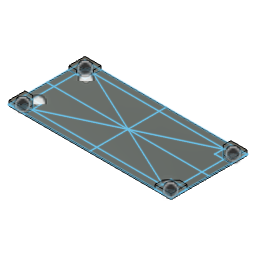
pcb_mount (Autodesk Fusion 360 design; units mm, degrees)
Autodesk Fusion 360 part; units mm, degrees
sketch "Sketch1" plane through (0, 0, 0) normal (0, 0, 1) x (1, 0, 0)
  line L0 (-1.15, -7.9615) -> (94.86, -7.9615)
  line L1 (94.86, -7.9615) -> (94.86, -52.9715)
  line L2 (94.86, -52.9715) -> (-1.15, -52.9715)
  line L3 (-1.15, -52.9715) -> (-1.15, -7.9615)
  line L4 (3, -11.9865) -> (90.71, -11.9865)
  line L5 (90.71, -11.9865) -> (90.71, -48.9465)
  line L6 (90.71, -48.9465) -> (3, -48.9465)
  line L7 (3, -48.9465) -> (3, -11.9865)
  line L8 (-1.15, -7.9615) -> (94.86, -52.9715)
  line L9 (94.86, -7.9615) -> (-1.15, -52.9715)
  line L10 (46.855, -30.4665) -> (46.855, -7.9615)
  line L11 (46.855, -30.4665) -> (46.855, -52.9715)
  line L12 (46.855, -30.4665) -> (94.86, -30.4665)
  line L13 (46.855, -30.4665) -> (-1.15, -30.4665)
  circle A0 centre (3, -11.9865) radius 1.55
  circle A1 centre (3, -48.9465) radius 1.55
  circle A2 centre (90.71, -48.9465) radius 1.55
  circle A3 centre (90.71, -11.9865) radius 1.55
  line L14 (6.2324, -12.0561) -> (4.6765, -9.2219)
  line L15 (4.6765, -9.2219) -> (1.4441, -9.1523)
  line L16 (1.4441, -9.1523) -> (-0.2324, -11.9168)
  line L17 (-0.2324, -11.9168) -> (1.3235, -14.751)
  line L18 (1.3235, -14.751) -> (4.5559, -14.8206)
  line L19 (4.5559, -14.8206) -> (6.2324, -12.0561)
  line L20 (4.6166, -51.7465) -> (6.2332, -48.9465)
  line L21 (6.2332, -48.9465) -> (4.6166, -46.1465)
  line L22 (4.6166, -46.1465) -> (1.3834, -46.1465)
  line L23 (1.3834, -46.1465) -> (-0.2332, -48.9465)
  line L24 (-0.2332, -48.9465) -> (1.3834, -51.7465)
  line L25 (1.3834, -51.7465) -> (4.6166, -51.7465)
  line L26 (92.3266, -51.7465) -> (93.9432, -48.9465)
  line L27 (93.9432, -48.9465) -> (92.3266, -46.1465)
  line L28 (92.3266, -46.1465) -> (89.0934, -46.1465)
  line L29 (89.0934, -46.1465) -> (87.4768, -48.9465)
  line L30 (87.4768, -48.9465) -> (89.0934, -51.7465)
  line L31 (89.0934, -51.7465) -> (92.3266, -51.7465)
  line L32 (92.3266, -14.7865) -> (93.9432, -11.9865)
  line L33 (93.9432, -11.9865) -> (92.3266, -9.1865)
  line L34 (92.3266, -9.1865) -> (89.0934, -9.1865)
  line L35 (89.0934, -9.1865) -> (87.4768, -11.9865)
  line L36 (87.4768, -11.9865) -> (89.0934, -14.7865)
  line L37 (89.0934, -14.7865) -> (92.3266, -14.7865)
  line L38 (-1.15, -7.9615) -> (8.35, -7.9615)
  line L39 (8.35, -7.9615) -> (8.35, -17.4615)
  line L40 (8.35, -17.4615) -> (-1.15, -17.4615)
  line L41 (-1.15, -17.4615) -> (-1.15, -7.9615)
  line L42 (3.3293, -17.4615) -> (8.35, -12.4407)
  line L43 (3.3293, -17.4615) -> (8.997, -17.4615) construction
  line L44 (-1.15, -52.9715) -> (8.35, -52.9715)
  line L45 (8.35, -52.9715) -> (8.35, -43.4715)
  line L46 (8.35, -43.4715) -> (-1.15, -43.4715)
  line L47 (-1.15, -43.4715) -> (-1.15, -52.9715)
  line L48 (3.3558, -43.4715) -> (8.35, -48.4657)
  line L49 (3.3558, -43.4715) -> (6.6655, -43.4715) construction
  line L50 (94.86, -52.9715) -> (85.36, -52.9715)
  line L51 (85.36, -52.9715) -> (85.36, -43.4715)
  line L52 (85.36, -43.4715) -> (94.86, -43.4715)
  line L53 (94.86, -43.4715) -> (94.86, -52.9715)
  line L54 (85.36, -48.4657) -> (90.3542, -43.4715)
  line L55 (85.36, -48.4657) -> (88.5571, -48.4657) construction
  line L56 (94.86, -7.9615) -> (85.36, -7.9615)
  line L57 (85.36, -7.9615) -> (85.36, -17.4615)
  line L58 (85.36, -17.4615) -> (94.86, -17.4615)
  line L59 (94.86, -17.4615) -> (94.86, -7.9615)
  line L60 (85.36, -12.4673) -> (90.3542, -17.4615)
  line L61 (85.36, -12.4673) -> (91.2896, -12.4673) construction
  point P0 (3, -11.9865)
  point P1 (3, -48.9465)
  point P2 (90.71, -48.9465)
  point P3 (90.71, -11.9865)
  dimension "d9" = 45.01
  dimension "d11" = 36.96
  dimension "d12" = 3.1
  dimension "d13" = 3.1
  dimension "d14" = 3.1
  dimension "d15" = 3.1
  dimension "d16" = 2.8
  dimension "d17" = 2.8
  dimension "d18" = 2.8
  dimension "d19" = 2.8
  dimension "d21" = 9.5
  dimension "d22" = 45
  dimension "d23" = 1
  dimension "d24" = 9.5
  dimension "d25" = 9.5
  dimension "d26" = 45
  dimension "d27" = 1
  dimension "d28" = 9.5
  dimension "d29" = 9.5
  dimension "d30" = 45
  dimension "d31" = 1
  dimension "d32" = 9.5
  dimension "d33" = 9.5
  dimension "d34" = 45
  dimension "d35" = 1
  constraint horizontal L0
  constraint vertical L1
  constraint horizontal L2
  constraint vertical L3
  constraint horizontal L4
  constraint vertical L5
  constraint horizontal L6
  constraint vertical L7
  constraint midpoint L9 L10.start
  constraint midpoint L0 L10.end
  constraint midpoint L2 L11.end
  constraint midpoint L1 L12.end
  constraint midpoint L3 L13.end
  constraint symmetric L4 L6 L12
  constraint symmetric L5 L7 L10
  constraint coincident P0 L4.start
  constraint coincident P1 L6.end
  constraint coincident P2 L5.end
  constraint coincident P3 L4.end
  constraint horizontal L38
  constraint vertical L39
  constraint horizontal L40
  constraint vertical L41
  constraint horizontal L43
  constraint coincident L40 L42.start
  constraint coincident L39 L42.end
  constraint horizontal L44
  constraint vertical L45
  constraint horizontal L46
  constraint vertical L47
  constraint horizontal L49
  constraint coincident L46 L48.start
  constraint coincident L45 L48.end
  constraint horizontal L50
  constraint vertical L51
  constraint horizontal L52
  constraint vertical L53
  constraint horizontal L55
  constraint coincident L51 L54.start
  constraint coincident L52 L54.end
  constraint horizontal L56
  constraint vertical L57
  constraint horizontal L58
  constraint vertical L59
  constraint horizontal L61
  constraint coincident L57 L60.start
  constraint coincident L58 L60.end
  measures "d9" distance of L0.start L2.end
  measures "d11" distance of P0 P1
  measures "d12" diameter of A0
  measures "d13" diameter of A1
  measures "d14" diameter of A2
  measures "d15" diameter of A3
  measures "d16" distance of P0 L19
  measures "d17" distance of P1 L25
  measures "d18" distance of P2 L31
  measures "d19" distance of P3 L37
  measures "d21" distance of L0.start L40.end
  measures "d22" angle of L42 L43
  measures "d23" distance of L18.end L42
  measures "d24" distance of L2.end L44.end
  measures "d25" distance of L2.end L46.end
  measures "d26" angle of L48 L49
  measures "d27" distance of L21.end L48
  measures "d28" distance of L1.end L50.end
  measures "d29" distance of L1.end L52.end
  measures "d30" angle of L54 L55
  measures "d31" distance of L28.end L54
  measures "d32" distance of L0.end L56.end
  measures "d33" distance of L0.end L58.end
  measures "d34" angle of L60 L61
  measures "d35" distance of L36.end L60
extrude "Extrude5" add sketch "Sketch1" against normal blind 0.8 contours L3 L7 L8 L16 L17 L18 L40 L41 | L0 L4 L8 L14 L15 L16 L38 L39 | L0 L4 L10 L39 | L3 L7 L13 L40 | L0 L4 L10 L57 | L4 L8 L39 | L4 L8 L10 L39 | L3 L7 L13 L46 | L7 L8 L13 L39 L40 | L4 L7 L8 L14 L18 L19 L39 L40 L42 | L4 L8 L14 | L0 L4 L9 L34 L35 L56 L57 | L4 L9 L10 L57 | L3 L7 L9 L22 L23 L24 L25 L46 L47 | L7 L9 L13 L45 L46 | L39 L40 L42 | L1 L5 L9 L32 L33 L34 L37 L58 L59 | L4 L9 L57 | L5 L8 L12 L51 L52 | L6 L9 L11 L45 | L6 L8 L11 L51 | L5 L9 L12 L57 L58 | L2 L6 L9 L20 L25 L44 L45 | L6 L7 L9 L21 L22 L45 L46 L48 | L1 L5 L12 L58 | L4 L9 L35 | L4 L5 L9 L36 L37 L57 L58 L60 | L5 L6 L8 L28 L29 L51 L52 L54 | L6 L8 L51 | L6 L9 L45 | L2 L6 L11 L45 | L2 L6 L11 L51 | L1 L5 L12 L52 | L45 L46 L48 | L57 L58 L60 | L2 L6 L8 L30 L31 L50 L51 | L6 L8 L30 | L51 L52 L54 | L6 L9 L20 | L1 L5 L8 L26 L27 L28 L31 L52 L53
extrude "Extrude6" add sketch "Sketch1" along normal blind 2.2 contours L3 L7 L8 L16 L17 L18 L40 L41 | L0 L4 L8 L14 L15 L16 L38 L39 | L4 L8 L39 | L4 L7 L8 L14 L18 L19 L39 L40 L42 | L4 L8 L14 | L0 L4 L9 L34 L35 L56 L57 | L3 L7 L9 L22 L23 L24 L25 L46 L47 | L1 L5 L9 L32 L33 L34 L37 L58 L59 | L4 L9 L57 | L2 L6 L9 L20 L25 L44 L45 | L6 L7 L9 L21 L22 L45 L46 L48 | L4 L9 L35 | L4 L5 L9 L36 L37 L57 L58 L60 | L5 L6 L8 L28 L29 L51 L52 L54 | L6 L8 L51 | L6 L9 L45 | L2 L6 L8 L30 L31 L50 L51 | L6 L8 L30 | L6 L9 L20 | L1 L5 L8 L26 L27 L28 L31 L52 L53
